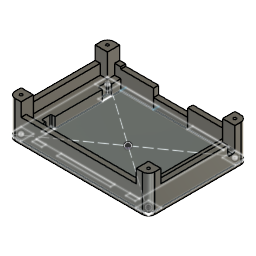
case base (Autodesk Fusion 360 design; units mm, degrees)
part number: 2026-07-02-10-34-18-857
Autodesk Fusion 360 part; units mm, degrees
note: some values were not read from the file. Chosen so that the rebuilt part matches the saved one: which bodies a step acts on.
sketch "Sketch1" plane through (0, 0, 0) normal (0, 0, 1) x (1, 0, 0)
  line L0 (68, -48) -> (-68, -48)
  line L1 (-68, -48) -> (-68, 48)
  line L2 (-68, 48) -> (68, 48)
  line L3 (68, 48) -> (68, -48)
  line L4 (68, -48) -> (-68, 48) construction
  line L5 (-68, -48) -> (68, 48) construction
  line L6 (-50, 43) -> (50, 43)
  line L7 (50, 43) -> (50, -39)
  line L8 (50, -39) -> (-50, -39)
  line L9 (-50, -39) -> (-50, 43)
  line L10 (-50, -39) -> (-41, -39)
  line L11 (-41, -39) -> (-41, -43)
  line L12 (-41, -43) -> (-50, -43)
  line L13 (-50, -43) -> (-50, -39)
  line L14 (50, -39) -> (41, -39)
  line L15 (41, -39) -> (41, -43)
  line L16 (41, -43) -> (50, -43)
  line L17 (50, -43) -> (50, -39)
  line L18 (-26, -39) -> (26, -39)
  line L19 (26, -39) -> (26, -43)
  line L20 (26, -43) -> (-26, -43)
  line L21 (-26, -43) -> (-26, -39)
  line L22 (-50, 34) -> (-54, 34)
  line L23 (-54, 34) -> (-54, 25)
  line L24 (-54, 25) -> (-50, 25)
  line L25 (-50, 25) -> (-50, 34)
  line L26 (-50, -30) -> (-54, -30)
  line L27 (-54, -30) -> (-54, -21)
  line L28 (-54, -21) -> (-50, -21)
  line L29 (-50, -21) -> (-50, -30)
  line L30 (68, 48) -> (56, 48)
  line L31 (56, 48) -> (56, 36)
  line L32 (56, 36) -> (68, 36)
  line L33 (68, 36) -> (68, 48)
  line L34 (-68, 48) -> (-56, 48)
  line L35 (-56, 48) -> (-56, 36)
  line L36 (-56, 36) -> (-68, 36)
  line L37 (-68, 36) -> (-68, 48)
  line L38 (68, -48) -> (56, -48)
  line L39 (56, -48) -> (56, -36)
  line L40 (56, -36) -> (68, -36)
  line L41 (68, -36) -> (68, -48)
  line L42 (-68, -48) -> (-56, -48)
  line L43 (-56, -48) -> (-56, -36)
  line L44 (-56, -36) -> (-68, -36)
  line L45 (-68, -36) -> (-68, -48)
  circle A0 centre (62, 42) radius 1.35
  circle A1 centre (-62, 42) radius 1.35
  circle A2 centre (-62, -42) radius 1.35
  circle A3 centre (62, -42) radius 1.35
  line L46 (-50.1525, 48) -> (-18.1525, 48)
  line L47 (-18.1525, 48) -> (-18.1525, 43)
  line L48 (-18.1525, 43) -> (-50.1525, 43)
  line L49 (-50.1525, 43) -> (-50.1525, 48)
  line L50 (50, 43) -> (15, 43)
  line L51 (15, 43) -> (15, 48)
  line L52 (15, 48) -> (50, 48)
  line L53 (50, 48) -> (50, 43)
  point P0 (62, -42)
  dimension "d3" = 136
  dimension "d4" = 96
  dimension "d5" = 100
  dimension "d6" = 82
  dimension "d7" = 5
  dimension "d8" = 18
  dimension "d9" = 9
  dimension "d10" = 4
  dimension "d11" = 9
  dimension "d12" = 4
  dimension "d13" = 4
  dimension "d14" = 15
  dimension "d15" = 15
  dimension "d16" = 4
  dimension "d17" = 9
  dimension "d18" = 9
  dimension "d19" = 4
  dimension "d20" = 9
  dimension "d21" = 9
  dimension "d24" = 12
  dimension "d25" = 12
  dimension "d26" = 12
  dimension "d27" = 12
  dimension "d28" = 12
  dimension "d29" = 12
  dimension "d30" = 12
  dimension "d31" = 12
  dimension "d32" = 2.7
  dimension "d33" = 6
  dimension "d34" = 6
  dimension "d35" = 2.7
  dimension "d36" = 2.7
  dimension "d37" = 2.7
  dimension "d38" = 6
  dimension "d39" = 6
  dimension "d40" = 6
  dimension "d41" = 6
  dimension "d42" = 6
  dimension "d43" = 6
  dimension "d44" = 32
  dimension "d45" = 5
  dimension "d46" = 35
  dimension "d47" = 5
  constraint horizontal L0
  constraint perpendicular L0 L1
  constraint parallel L0 L2
  constraint parallel L1 L3
  constraint coincident L4 origin
  constraint coincident L5 origin
  constraint horizontal L6
  constraint vertical L7
  constraint horizontal L8
  constraint vertical L9
  constraint horizontal L10
  constraint vertical L11
  constraint horizontal L12
  constraint vertical L13
  constraint horizontal L14
  constraint vertical L15
  constraint horizontal L16
  constraint vertical L17
  constraint horizontal L18
  constraint vertical L19
  constraint horizontal L20
  constraint vertical L21
  constraint coincident L8 L18.start
  constraint horizontal L22
  constraint vertical L23
  constraint horizontal L24
  constraint vertical L25
  constraint coincident L9 L22.start
  constraint horizontal L26
  constraint vertical L27
  constraint horizontal L28
  constraint vertical L29
  constraint coincident L9 L26.start
  constraint horizontal L30
  constraint vertical L31
  constraint horizontal L32
  constraint vertical L33
  constraint horizontal L34
  constraint vertical L35
  constraint horizontal L36
  constraint vertical L37
  constraint horizontal L38
  constraint vertical L39
  constraint horizontal L40
  constraint vertical L41
  constraint horizontal L42
  constraint vertical L43
  constraint horizontal L44
  constraint vertical L45
  constraint coincident P0 A3.centre
  constraint horizontal L46
  constraint vertical L47
  constraint horizontal L48
  constraint vertical L49
  constraint coincident L2 L46.start
  constraint horizontal L50
  constraint vertical L51
  constraint horizontal L52
  constraint vertical L53
  measures "d3" distance of L1.end L2.end
  measures "d4" distance of L0.end L1.end
  measures "d5" distance of L6.start L6.end
  measures "d6" distance of L6.start L8.end
  measures "d7" distance of L2 L6
  measures "d8" distance of L3 L7
  measures "d9" distance of L8.end L10.end
  measures "d10" distance of L8.end L12.end
  measures "d11" distance of L7.end L14.end
  measures "d12" distance of L7.end L16.end
  measures "d13" distance of L18.start L20.end
  measures "d14" distance of L11 L21
  measures "d15" distance of L15 L19
  measures "d16" distance of L22.start L22.end
  measures "d17" distance of L22.start L24.end
  measures "d18" distance of L6 L22
  measures "d19" distance of L26.start L26.end
  measures "d20" distance of L26.start L28.end
  measures "d21" distance of L10 L26
  measures "d24" distance of L2.end L30.end
  measures "d25" distance of L2.end L32.end
  measures "d26" distance of L1.end L34.end
  measures "d27" distance of L1.end L36.end
  measures "d28" distance of L0.start L38.end
  measures "d29" distance of L0.start L40.end
  measures "d30" distance of L0.end L42.end
  measures "d31" distance of L0.end L44.end
  measures "d32" diameter of A0
  measures "d33" distance of L31 A0.centre
  measures "d34" distance of L30 A0.centre
  measures "d35" diameter of A1
  measures "d36" diameter of A2
  measures "d37" diameter of A3
  measures "d38" distance of L41 P0
  measures "d39" distance of L38 P0
  measures "d40" distance of L44 A2.centre
  measures "d41" distance of L45 A2.centre
  measures "d42" distance of L34 A1.centre
  measures "d43" distance of L37 A1.centre
  measures "d44" distance of L46.start L46.end
  measures "d45" distance of L46.start L48.end
  measures "d46" distance of L6.end L50.end
  measures "d47" distance of L6.end L52.end
extrude "Extrude1" add sketch "Sketch1" against normal blind 3 contours L0 L3 L38 L39 L40 L41 | L0 L1 L2 L3 L7 L8 L9 L11 L12 L13 L15 L16 L17 L19 L20 L21 L22 L23 L24 L26 L27 L28 L31 L32 L35 L36 L39 L40 L43 L44 L48 L49 L53 | L0 L1 L42 L43 L44 L45 | L2 L3 L30 L31 L32 L33 | L1 L2 L34 L35 L36 L37 | L2 L6 L50 L51 L52 L53 | L2 L6 L47 L51 | L6 L7 L8 L9 L10 L14 L18 L25 L29 L48 L50 | L2 L6 L46 L47 L48 L49 | L8 L14 L15 L16 L17 | L8 L18 L19 L20 L21 | L9 L22 L23 L24 L25 | L8 L10 L11 L12 L13 | L9 L26 L27 L28 L29 | A0 | A1 | A2 | A3 makes body 1
extrude "Extrude2" add sketch "Sketch1" along normal blind 33 separate body contours L0 L3 L38 L39 L40 L41 | L0 L1 L42 L43 L44 L45 | L2 L3 L30 L31 L32 L33 | L1 L2 L34 L35 L36 L37 makes body 2 at (60, 36, 22) makes body 3 at (60, -36, 22) makes body 4 at (-60, 36, 22) makes body 5 at (-60, -36, 22)
extrude "Extrude3" add sketch "Sketch1" against normal blind 3 separate body contours A0 | A1 | A2 | A3 makes body 6 at (-63.3433, 41.8656, -2) makes body 7 at (60.6567, 41.8656, -2) makes body 8 at (-63.3433, -42.1344, -2) makes body 9 at (60.6567, -42.1344, -2)
extrude "Extrude4" cut sketch "Sketch1" against normal blind 3 contours A0 bodies 1 7
extrude "Extrude5" cut sketch "Sketch1" against normal blind 3 contours A1 bodies 1 6
extrude "Extrude6" cut sketch "Sketch1" against normal blind 3 contours A3 bodies 1 9
extrude "Extrude7" cut sketch "Sketch1" against normal blind 3 contours A2 bodies 1 8
extrude "Extrude8" add sketch "Sketch1" along normal blind 10 separate body contours L0 L1 L2 L3 L7 L8 L9 L11 L12 L13 L15 L16 L17 L19 L20 L21 L22 L23 L24 L26 L27 L28 L31 L32 L35 L36 L39 L40 L43 L44 L48 L49 L53 | L2 L6 L47 L51 makes body 10 at (-63.3333, -7, 0) makes body 11 at (-7.1017, 43, 3.3333)
fillet "Fillet1" radius 6 8 edges at (-68, -48, -1.5) (68, -48, -1.5) (68, 48, -1.5) (-68, 48, -1.5) (68, 48, 16.5) (68, -48, 16.5) (-68, 48, 16.5) (-68, -48, 16.5) on bodies 1 2 3 4 5
extrude "Extrude9" add sketch "Sketch1" along normal blind 18 separate body contours L2 L6 L50 L51 L52 L53 | L2 L6 L46 L47 L48 L49 makes body 12 at (-39.4858, 43, 6) makes body 13 at (26.6667, 43, 6)
sketch "Sketch2" plane through (0, 0, 10) normal (0, 0, 1) x (-1, 0, 0)
  line L0 (-56, -48) -> (-50, -48)
  line L1 (-50, -48) -> (-50, 43)
  line L2 (-50, 43) -> (-41, 43)
  line L3 (-41, 43) -> (-41, 39)
  line L4 (-41, 39) -> (-26, 39)
  line L5 (-26, 39) -> (-26, 43)
  line L6 (-26, 43) -> (26, 43)
  line L7 (26, 43) -> (26, 39)
  line L8 (26, 39) -> (41, 39)
  line L9 (41, 39) -> (41, 43)
  line L10 (41, 43) -> (50, 43)
  line L11 (50, 43) -> (50, 30)
  line L12 (50, 30) -> (54, 30)
  line L13 (54, 30) -> (54, 21)
  line L14 (54, 21) -> (50, 21)
  line L15 (50, 21) -> (50, -25)
  line L16 (50, -25) -> (54, -25)
  line L17 (54, -25) -> (54, -34)
  line L18 (54, -34) -> (50, -34)
  line L19 (50, -34) -> (50, -43)
  line L20 (50, -43) -> (50.1525, -43)
  line L21 (50.1525, -43) -> (50.1525, -48)
  line L22 (50.1525, -48) -> (56, -48)
  line L23 (56, -48) -> (56, -36)
  line L24 (56, -36) -> (68, -36)
  line L25 (68, -36) -> (68, 36)
  line L26 (68, 36) -> (56, 36)
  line L27 (56, 36) -> (56, 48)
  line L28 (56, 48) -> (-56, 48)
  line L29 (-56, 48) -> (-56, 36)
  line L30 (-56, 36) -> (-68, 36)
  line L31 (-68, 36) -> (-68, -36)
  line L32 (-68, -36) -> (-56, -36)
  line L33 (-56, -36) -> (-56, -48)
  line L34 (-68, -36) -> (-50, -36)
  line L35 (-50, -36) -> (-50, -29)
  line L36 (-50, -29) -> (-68, -29)
  line L37 (-68, -29) -> (-68, -36)
  line L38 (-56, -48) -> (-50, -48)
  line L39 (-50, -48) -> (-50, -43)
  line L40 (-50, -43) -> (-56, -43)
  line L41 (-56, -43) -> (-56, -48)
  line L42 (-68, -29) -> (-63, -29)
  line L43 (-63, -29) -> (-63, 36)
  line L44 (-63, 36) -> (-68, 36)
  line L45 (-68, 36) -> (-68, -29)
  line L46 (-56, 48) -> (56, 48)
  line L47 (56, 48) -> (56, 43)
  line L48 (56, 43) -> (-56, 43)
  line L49 (-56, 43) -> (-56, 48)
  line L50 (68, -36) -> (63, -36)
  line L51 (63, -36) -> (63, 36)
  line L52 (63, 36) -> (68, 36)
  line L53 (68, 36) -> (68, -36)
  line L54 (50, -43) -> (56, -43)
  line L55 (56, -43) -> (56, -48)
  line L56 (56, -48) -> (50, -48)
  line L57 (50, -48) -> (50, -43)
  line L58 (68, 36) -> (63, 36)
  line L59 (63, 36) -> (63, 30.6)
  line L60 (63, 30.6) -> (68, 30.6)
  line L61 (68, 30.6) -> (68, 36)
  dimension "d66" = 7
  dimension "d67" = 5
  dimension "d68" = 5
  dimension "d69" = 5
  dimension "d70" = 5.4
  constraint horizontal L34
  constraint vertical L35
  constraint horizontal L36
  constraint vertical L37
  constraint coincident L31.end L32.start
  constraint horizontal L38
  constraint vertical L39
  constraint horizontal L40
  constraint vertical L41
  constraint coincident L1 L39.end
  constraint coincident L0.start L33.end
  constraint horizontal L42
  constraint vertical L43
  constraint horizontal L44
  constraint vertical L45
  constraint horizontal L46
  constraint vertical L47
  constraint horizontal L48
  constraint vertical L49
  constraint coincident L27 L47.end
  constraint coincident L28.end L29.start
  constraint horizontal L50
  constraint vertical L51
  constraint horizontal L52
  constraint vertical L53
  constraint coincident L24.end L25.start
  constraint horizontal L54
  constraint vertical L55
  constraint horizontal L56
  constraint vertical L57
  constraint coincident L22.end L23.start
  constraint coincident L19.end L20.start
  constraint horizontal L58
  constraint vertical L59
  constraint horizontal L60
  constraint vertical L61
  constraint coincident L25.end L26.start
  measures "d66" distance of L31.end L36.end
  measures "d67" distance of L36.end L42.end
  measures "d68" distance of L24.end L50.end
  measures "d69" distance of L25.end L51.end
  measures "d70" distance of L25.end L60.end
extrude "Extrude10" add sketch "Sketch2" along normal blind 10 contours L0 L1 L33 L38 L39 L40 L41 | L30 L31 L36 L42 L43 L44 L45 | L2 L6 L10 L27 L28 L29 L46 L47 L48 L49 | L24 L25 L50 L51 L53 L60 | L21 L22 L23 L54 L55 L56 bodies 1 2 11 3 4 5 10 12 13
fillet "Fillet2" radius 1 4 edges at (-54, 34, 5) (-54, 25, 5) (-54, -30, 5) (-54, -21, 5) on bodies 2
fillet "Fillet3" radius 1 2 edges at (50, -43, 5) (41, -43, 5) on bodies 2
fillet "Fillet4" radius 1 2 edges at (26, -43, 5) (-26, -43, 5) on bodies 2
fillet "Fillet5" radius 1 2 edges at (-41, -43, 5) (-50, -43, 5) on bodies 2
fillet "Fillet6" radius 2 2 edges at (65.5, 29, 10) (62, 36, 10) on bodies 2
